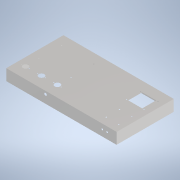
# Autodesk Inventor part: Gehaeuse_Deckel
Saved by Autodesk Inventor 2020 (Build 240168000, 168)
## iProperties
Created: 2019-01-15
Part Number: Gehaeuse_Deckel
Material: Generic
Document SubType Name: Modeling
Designer: patri
Density: 1 g/cm^3
Appearance: Aluminum - Dark
Author: Patrik Staudenmayer
Autodesk Inventor part; units mm, degrees
ref_plane "YZ Plane" through (0, 0, 0) normal (1, 0, 0) x (0, 1, 0)
ref_plane "XZ Plane" through (0, 0, 0) normal (0, 1, 0) x (-1, 0, 0)
ref_plane "XY Plane" through (0, 0, 0) normal (0, 0, 1) x (1, 0, 0)
sketch "Sketch1" plane through (0, 0, 0) normal (0, 1, 0) x (-1, 0, 0)
  line L0 (222, -115) -> (-222, -115)
  line L1 (-222, -115) -> (-222, 115)
  line L2 (-222, 115) -> (222, 115)
  line L3 (222, 115) -> (222, -115)
  line L4 (0, -161) -> (0, 161) projected
  line L5 (310.8, 0) -> (-310.8, 0) projected
  point P0 (0, 0)
  dimension "d0" = 444
  dimension "d1" = 230
  constraints: 8 end point, 2 parallel, 1 horizontal, 1 perpendicular, 2 other
  measures "d0" distance of L0.start L0.end
  measures "d1" distance of L0.end L1.end
extrude "Extrusion1" add sketch "Sketch1" along normal blind 45
sketch "Sketch10" plane through (0, 0, 0) normal (0, -1, 0) x (1, 0, 0)
  line L0 (-221.88, 114.88) -> (221.88, 114.88)
  line L1 (221.88, 114.88) -> (221.88, -114.88)
  line L2 (221.88, -114.88) -> (-221.88, -114.88)
  line L3 (-221.88, -114.88) -> (-221.88, 114.88)
  line L4 (0, -161) -> (0, 161) projected
  line L5 (-310.8, 0) -> (310.8, 0) projected
  line L6 (-222, 115) -> (-222, -115) projected
  line L7 (222, 115) -> (-222, 115) projected
  point P0 (0, 0)
  dimension "d19" = 0.12
  dimension "d20" = 0.12
  constraints: 8 end point, 2 parallel, 1 horizontal, 1 perpendicular, 2 other
  measures "d19" distance between parallel lines of L3 L6
  measures "d20" distance between parallel lines of L0 L7
extrude "Extrusion6" cut sketch "Sketch10" against normal blind 44.88 contours L0 L4 L5 L3 | L0 L1 L5 L4 | L5 L4 L2 L3 | L5 L1 L2 L4
sketch "Sketch11" plane through (0, 45, 0) normal (0, 1, 0) x (1, 0, 0)
  circle A0 centre (-189, -70) radius 11
  line L0 (-222, 115) -> (-222, -115) projected
  line L1 (-222, -115) -> (222, -115) projected
  circle A1 centre (-125, -70) radius 11
  circle A2 centre (-61, -70) radius 11
  line L2 (-221.88, 114.88) -> (-221.88, -114.88) projected
  line L3 (-221.88, -70) -> (1.88, -70) construction
  circle A3 centre (-174, -70) radius 2
  circle A4 centre (-204, -70) radius 2
  circle A5 centre (-140, -70) radius 2
  circle A6 centre (-110, -70) radius 2
  circle A7 centre (-76, -70) radius 2
  circle A8 centre (-46, -70) radius 2
  line L4 (-60.23, 75.55) -> (-189.48, 75.55) construction
  line L5 (-189.48, 75.55) -> (-189.48, -16.15) construction
  line L6 (-189.48, -16.15) -> (-60.23, -16.15) construction
  line L7 (-60.23, -16.15) -> (-60.23, 75.55) construction
  line L8 (222, 115) -> (-222, 115) projected
  circle A9 centre (-189.48, 75.55) radius 2
  circle A10 centre (-60.23, 75.55) radius 2
  circle A11 centre (-60.23, -16.15) radius 2
  circle A12 centre (-189.48, -16.15) radius 2
  point P0 (0, 0)
  dimension "d24" = 22
  dimension "d25" = 33
  dimension "d27" = 22
  dimension "d30" = 64
  dimension "d31" = 22
  dimension "d33" = 64
  dimension "d35" = 45
  dimension "d36" = 4
  dimension "d37" = 15
  dimension "d38" = 4
  dimension "d39" = 15
  dimension "d40" = 4
  dimension "d41" = 4
  dimension "d42" = 4
  dimension "d43" = 4
  dimension "d44" = 15
  dimension "d45" = 15
  dimension "d46" = 15
  dimension "d47" = 15
  dimension "d50" = 129.25
  dimension "d52" = 39.45
  dimension "d54" = 32.4
  dimension "d55" = 91.7
  dimension "d56" = 4
  dimension "d57" = 4
  dimension "d58" = 4
  dimension "d59" = 4
  constraints: 13 centre point, 8 end point, 4 coincident, 2 horizontal, 2 parallel, 1 perpendicular, 1 point on line, 12 other
  measures "d24" diameter of A0
  measures "d25" distance from line of L0 A0.centre
  measures "d27" diameter of A1
  measures "d30" distance of A0.centre A1.centre
  measures "d31" diameter of A2
  measures "d33" distance of A1.centre A2.centre
  measures "d36" diameter of A3
  measures "d37" distance of A0.centre A3.centre
  measures "d38" diameter of A4
  measures "d39" distance of A0.centre A4.centre
  measures "d40" diameter of A5
  measures "d41" diameter of A6
  measures "d42" diameter of A7
  measures "d43" diameter of A8
  measures "d44" distance of A5.centre A1.centre
  measures "d45" distance of A1.centre A6.centre
  measures "d46" distance of A2.centre A7.centre
  measures "d47" distance of A8.centre A2.centre
  measures "d50" distance of L4.start L4.end
  measures "d52" distance between parallel lines of L8 L4
  measures "d54" distance between parallel lines of L2 L5
  measures "d55" distance of L6.end L4.start
  measures "d56" diameter of A9
  measures "d57" diameter of A10
  measures "d58" diameter of A11
  measures "d59" diameter of A12
extrude "Extrusion7" cut sketch "Sketch11" against normal up to next
sketch "Sketch12" plane through (0, 45, 0) normal (0, 1, 0) x (1, 0, 0)
  line L0 (129, 74.35) -> (199.5, 74.35) construction
  line L1 (199.5, 74.35) -> (199.5, 18.35) construction
  line L2 (199.5, 18.35) -> (129, 18.35) construction
  line L3 (129, 18.35) -> (129, 74.35) construction
  line L4 (222, 115) -> (-222, 115) projected
  line L5 (199.5, 115) -> (199.5, -115) construction
  line L6 (-222, -115) -> (222, -115) projected
  line L7 (222, -115) -> (222, 115) projected
  circle A0 centre (129, 74.35) radius 2.1
  circle A1 centre (199.5, 74.35) radius 2.1
  circle A2 centre (199.5, 18.35) radius 2.1
  circle A3 centre (129, 18.35) radius 2.1
  point P0 (0, 0)
  dimension "d65" = 22.5
  dimension "d66" = 40.65
  dimension "d67" = 56
  dimension "d68" = 4.2
  dimension "d69" = 4.2
  dimension "d70" = 4.2
  dimension "d71" = 4.2
  dimension "d72" = 70.5
  constraints: 10 end point, 4 centre point, 4 coincident, 3 parallel, 3 point on line, 1 horizontal, 1 perpendicular, 1 vertical
  measures "d65" distance between parallel lines of L7 L5
  measures "d66" distance between parallel lines of L4 L0
  measures "d67" distance of L2.end L0.start
  measures "d68" diameter of A0
  measures "d69" diameter of A1
  measures "d70" diameter of A2
  measures "d71" diameter of A3
  measures "d72" distance of L0.start L0.end
extrude "Extrusion8" cut sketch "Sketch12" against normal up to next
sketch "Sketch13" plane through (0, 45, 0) normal (0, 1, 0) x (1, 0, 0)
  line L0 (149.8, -31.1) -> (199.5, -31.1) construction
  line L1 (199.5, -31.1) -> (199.5, -84.5) construction
  line L2 (199.5, -84.5) -> (149.8, -84.5) construction
  line L3 (149.8, -84.5) -> (149.8, -31.1) construction
  line L4 (222, -115) -> (222, 115) projected
  line L5 (-222, -115) -> (222, -115) projected
  line L6 (199.5, 74.35) -> (199.5, 18.35) construction
  line L7 (199.5, 115) -> (199.5, -115) construction
  circle A0 centre (199.5, -31.1) radius 2.1
  circle A1 centre (149.8, -31.1) radius 2.1
  circle A2 centre (149.8, -84.5) radius 2.1
  circle A3 centre (199.5, -84.5) radius 2.1
  point P0 (0, 0)
  dimension "d75" = 49.7
  dimension "d77" = 53.4
  dimension "d79" = 30.5
  dimension "d80" = 4.2
  dimension "d81" = 4.2
  dimension "d82" = 4.2
  dimension "d83" = 4.2
  constraints: 8 end point, 4 centre point, 4 coincident, 2 parallel, 1 horizontal, 1 perpendicular, 1 point on line
  measures "d75" distance of L0.start L0.end
  measures "d77" distance of L2.end L0.start
  measures "d79" distance between parallel lines of L5 L2
  measures "d80" diameter of A0
  measures "d81" diameter of A1
  measures "d82" diameter of A2
  measures "d83" diameter of A3
extrude "Extrusion9" cut sketch "Sketch13" against normal up to next
sketch "Sketch14" plane through (0, 45, 0) normal (0, 1, 0) x (1, 0, 0)
  line L0 (199.5, 74.35) -> (199.5, 18.35) construction
  line L1 (129, 74.35) -> (199.5, 74.35) construction
  line L2 (199.5, 18.35) -> (129, 18.35) construction
  line L3 (129, 18.35) -> (129, 74.35) construction
  line L4 (135.6, 74.35) -> (191.6, 74.35)
  line L5 (191.6, 74.35) -> (191.6, 18.35)
  line L6 (191.6, 18.35) -> (135.6, 18.35)
  line L7 (135.6, 18.35) -> (135.6, 74.35)
  line L8 (121.9, 81.45) -> (206.6, 81.45) construction
  line L9 (206.6, 81.45) -> (206.6, 11.25) construction
  line L10 (206.6, 11.25) -> (121.9, 11.25) construction
  line L11 (121.9, 11.25) -> (121.9, 81.45) construction
  point P0 (0, 0)
  dimension "d86" = 56
  dimension "d87" = 56
  dimension "d88" = 7.1
  dimension "d89" = 7.1
  dimension "d90" = 7.1
  dimension "d92" = 15
  dimension "d94" = 7.1
  constraints: 16 end point, 4 parallel, 2 horizontal, 2 perpendicular, 1 point on line
  measures "d86" distance of L4.start L4.end
  measures "d87" distance of L6.end L4.start
  measures "d88" distance between parallel lines of L8 L1
  measures "d89" distance between parallel lines of L10 L2
  measures "d90" distance between parallel lines of L9 L0
  measures "d92" distance between parallel lines of L9 L5
  measures "d94" distance between parallel lines of L11 L3
extrude "Extrusion10" cut sketch "Sketch14" against normal up to next
sketch "Sketch16" plane through (-222, 0, 115) normal (0, 0, 1) x (1, 0, 0)
  circle A0 centre (406, 25) radius 3
  line L0 (444, 0) -> (444, 45) projected
  line L1 (444, 0) -> (0, 0) projected
  circle A1 centre (386.6, 25) radius 3
  line L2 (443.88, 0) -> (443.88, 44.88) projected
  line L3 (443.88, 25) -> (334.929, 25) construction
  point P0 (222, 0)
  dimension "d97" = 6
  dimension "d98" = 38
  dimension "d100" = 6
  dimension "d101" = 108.951
  dimension "d102" = 25
  dimension "d103" = 19.4
  constraints: 3 point on line, 2 centre point, 2 end point, 1 horizontal
  measures "d97" diameter of A0
  measures "d98" distance from line of L0 A0.centre
  measures "d100" diameter of A1
  measures "d101" distance of L3.start L3.end
  measures "d102" distance between parallel lines of L1 L3
  measures "d103" distance of A0.centre A1.centre
extrude "Extrusion11" cut sketch "Sketch16" against normal up to surface (0.12 mm away)
sketch "Sketch17" plane through (-222, 0, 115) normal (0, 0, 1) x (1, 0, 0)
  circle A0 centre (158, 33) radius 5
  line L0 (0, 0) -> (0, 45) projected
  line L1 (444, 0) -> (0, 0) projected
  point P0 (222, 0)
  dimension "d106" = 10
  dimension "d107" = 158
  dimension "d108" = 33
  constraints: 1 centre point
  measures "d106" diameter of A0
  measures "d107" distance from line of L0 A0.centre
  measures "d108" distance from line of L1 A0.centre
extrude "Extrusion12" cut sketch "Sketch17" against normal up to surface (0.12 mm away)
sketch "Sketch18" plane through (222, 0, -115) normal (0, 0, -1) x (-1, 0, 0)
  line L0 (19, 40.5) -> (32, 40.5)
  line L1 (32, 40.5) -> (32, 10.5)
  line L2 (32, 10.5) -> (19, 10.5)
  line L3 (19, 10.5) -> (19, 40.5)
  line L4 (19, 40.5) -> (32, 10.5) construction
  line L5 (32, 40.5) -> (19, 10.5) construction
  line L6 (0, 45) -> (444, 45) projected
  line L7 (0, 0) -> (0, 45) projected
  point P0 (222, 0)
  point P1 (25.5, 25.5)
  dimension "d111" = 13
  dimension "d112" = 30
  dimension "d113" = 4.5
  dimension "d114" = 19
  constraints: 12 end point, 2 midpoint, 2 parallel, 1 horizontal, 1 perpendicular
  measures "d111" distance of L0.start L0.end
  measures "d112" distance of L2.end L0.start
  measures "d113" distance between parallel lines of L6 L0
  measures "d114" distance between parallel lines of L7 L3
extrude "Extrusion13" cut sketch "Sketch18" against normal up to surface (0.12 mm away)
sketch "Sketch19" plane through (222, 0, -115) normal (0, 0, -1) x (-1, 0, 0)
  circle A0 centre (371.75, 32) radius 4.25
  line L0 (444, 0) -> (444, 45) projected
  line L1 (444, 32) -> (305.1223, 32) construction
  line L2 (444, 0) -> (0, 0) projected
  circle A1 centre (347.15, 32) radius 4.25
  line L3 (0, 45) -> (444, 45) projected
  point P0 (222, 0)
  dimension "d117" = 8.5
  dimension "d118" = 138.8777
  dimension "d120" = 72.25
  dimension "d121" = 8.5
  dimension "d122" = 24.6
  dimension "d123" = 13
  constraints: 3 point on line, 2 centre point, 2 end point, 1 horizontal
  measures "d117" diameter of A0
  measures "d118" distance of L1.start L1.end
  measures "d120" distance from line of L0 A0.centre
  measures "d121" diameter of A1
  measures "d122" distance of A0.centre A1.centre
  measures "d123" distance between parallel lines of L3 L1
extrude "Extrusion14" cut sketch "Sketch19" against normal up to surface (0.12 mm away)
sketch "Sketch20" plane through (222, 0, -115) normal (0, 0, -1) x (-1, 0, 0)
  line L0 (218, 28) -> (270, 28)
  line L1 (270, 28) -> (270, 11)
  line L2 (270, 11) -> (218, 11)
  line L3 (218, 11) -> (218, 28)
  line L4 (218, 28) -> (270, 11) construction
  line L5 (270, 28) -> (218, 11) construction
  line L6 (0, 45) -> (444, 45) projected
  line L7 (182.7735, 19.5) -> (305.684, 19.5) construction
  line L8 (444, 0) -> (444, 45) projected
  circle A0 centre (213, 19.5) radius 2
  circle A1 centre (275, 19.5) radius 2
  line L9 (244, 36.5338) -> (244, 7.8411) construction
  point P0 (222, 0)
  point P1 (244, 19.5)
  point P2 (244, 19.5)
  point P3 (244, 19.5)
  dimension "d126" = 52
  dimension "d127" = 17
  dimension "d129" = 17
  dimension "d130" = 200
  dimension "d131" = 4
  dimension "d132" = 4
  dimension "d133" = 5
  constraints: 16 end point, 4 midpoint, 4 point on line, 2 centre point, 2 horizontal, 2 parallel, 1 perpendicular, 1 symmetric about line, 1 vertical
  measures "d126" distance of L0.start L0.end
  measures "d127" distance of L0.end L1.end
  measures "d129" distance between parallel lines of L6 L0
  measures "d130" distance from line of L8 point (244, 19.5)
  measures "d131" diameter of A0
  measures "d132" diameter of A1
  measures "d133" distance from line of L3 A0.centre
extrude "Extrusion15" cut sketch "Sketch20" against normal up to surface (0.12 mm away)
equation "\"d60\" = d56"
equation "\"d95\" = d56"
body "Solid1"
